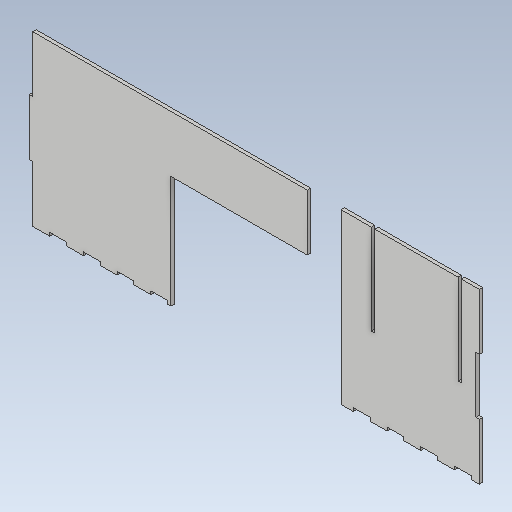
# Autodesk Inventor part: ParedFrontal
Saved by Autodesk Inventor 2020 (Build 240168000, 168)
## iProperties
Created: 2020-03-08
Part Number: ParedFrontal
Material: Genérico
Document SubType Name: Modeling
Designer: Diego Guillén
Density: 1 g/cm^3
Appearance: Valor por defecto
Author: Diego Guillén
Autodesk Inventor part; units mm, degrees
ref_plane "YZ Plane" through (0, 0, 0) normal (1, 0, 0) x (0, 1, 0)
ref_plane "XZ Plane" through (0, 0, 0) normal (0, 1, 0) x (-1, 0, 0)
ref_plane "XY Plane" through (0, 0, 0) normal (0, 0, 1) x (1, 0, 0)
sketch "Boceto1" plane through (0, 0, 0) normal (0, 0, 1) x (1, 0, 0)
  line L0 (0, 0) -> (400, 0)
  line L1 (400, 0) -> (400, 150)
  line L2 (400, 150) -> (0, 150)
  line L3 (0, 150) -> (0, 0)
  dimension "d0" = 150
  dimension "d1" = 400
  constraints: 8 end point, 2 parallel, 1 horizontal, 1 perpendicular
  measures "d0" distance of L0.end L1.end
  measures "d1" distance of L1.end L2.end
extrude "Extrusión1" add sketch "Boceto1" along normal blind 3
sketch "Boceto3" plane through (0, 0, 3) normal (0, 0, 1) x (1, 0, 0)
  line L0 (0, 0) -> (400, 0) construction
  line L1 (400, 0) -> (400, 150) construction
  line L2 (400, 150) -> (0, 150) construction
  line L3 (0, 150) -> (0, 0) construction
  line L4 (0, 50) -> (3, 50)
  line L5 (3, 50) -> (3, 0)
  line L6 (3, 0) -> (0, 0)
  line L7 (0, 0) -> (0, 50)
  line L8 (0, 100) -> (0, 150)
  line L9 (0, 150) -> (3, 150)
  line L10 (3, 150) -> (3, 100)
  line L11 (3, 100) -> (0, 100)
  line L12 (397, 100) -> (400, 100)
  line L13 (400, 100) -> (400, 50)
  line L14 (400, 50) -> (397, 50)
  line L15 (397, 50) -> (397, 100)
  line L16 (400, 0) -> (400, 150) construction
  point P0 (400, 75)
  point P1 (400, 75)
  dimension "d15" = 3
  dimension "d16" = 50
  dimension "d19" = 100
  dimension "d24" = 3
  dimension "d25" = 50
  constraints: 24 end point, 4 parallel, 2 coincident, 2 horizontal, 2 midpoint, 2 perpendicular, 1 collinear, 1 vertical, 8 other
  measures "d15" distance of L5.end L6.end
  measures "d16" distance of L4.end L5.end
  measures "d19" distance of L6.end L8.start
  measures "d24" distance of L13.end L14.end
  measures "d25" distance of L14.end L12.start
extrude "Extrusión3" cut sketch "Boceto3" against normal blind 3
sketch "Boceto4" plane through (0, 0, 3) normal (0, 0, 1) x (1, 0, 0)
  line L0 (3, 150) -> (3, 100) construction
  line L1 (3, 100) -> (0, 100) construction
  line L2 (0, 100) -> (0, 50) construction
  line L3 (0, 50) -> (3, 50) construction
  line L4 (3, 50) -> (3, 0) construction
  line L5 (3, 0) -> (400, 0) construction
  line L6 (400, 0) -> (400, 50) construction
  line L7 (400, 50) -> (397, 50) construction
  line L8 (397, 50) -> (397, 100) construction
  line L9 (397, 100) -> (400, 100) construction
  line L10 (400, 100) -> (400, 150) construction
  line L11 (400, 150) -> (3, 150) construction
  line L12 (277.1, 100) -> (125.9, 100)
  line L13 (125.9, 100) -> (125.9, 0)
  line L14 (125.9, 0) -> (277.1, 0)
  line L15 (277.1, 0) -> (277.1, 100)
  line L16 (3, 0) -> (400, 0) construction
  point P0 (0, 0)
  point P1 (201.5, 0)
  point P2 (201.5, 0)
  dimension "d28" = 151.2
  dimension "d29" = 100
  constraints: 8 end point, 2 midpoint, 2 parallel, 1 coincident, 1 collinear, 1 horizontal, 1 perpendicular
  measures "d28" distance of L12.start L12.end
  measures "d29" distance of L14.end L12.start
extrude "Extrusión4" cut sketch "Boceto4" against normal blind 10
sketch "Boceto5" plane through (0, 0, 3) normal (0, 0, 1) x (1, 0, 0)
  line L0 (277.1, 100) -> (277.1, 0) construction
  line L1 (277.1, 0) -> (400, 0) construction
  line L2 (400, 0) -> (400, 50) construction
  line L3 (400, 50) -> (397, 50) construction
  line L4 (397, 50) -> (397, 100) construction
  line L5 (397, 100) -> (400, 100) construction
  line L6 (400, 100) -> (400, 150) construction
  line L7 (400, 150) -> (3, 150) construction
  line L8 (3, 150) -> (3, 100) construction
  line L9 (3, 100) -> (0, 100) construction
  line L10 (0, 100) -> (0, 50) construction
  line L11 (0, 50) -> (3, 50) construction
  line L12 (3, 50) -> (3, 0) construction
  line L13 (3, 0) -> (125.9, 0) construction
  line L14 (125.9, 0) -> (125.9, 100) construction
  line L15 (125.9, 100) -> (277.1, 100) construction
  line L16 (304.1, 150) -> (307.1, 150)
  line L17 (307.1, 150) -> (307.1, 70)
  line L18 (307.1, 70) -> (304.1, 70)
  line L19 (304.1, 70) -> (304.1, 150)
  line L20 (381.1, 150) -> (384.1, 150)
  line L21 (384.1, 150) -> (384.1, 70)
  line L22 (384.1, 70) -> (381.1, 70)
  line L23 (381.1, 70) -> (381.1, 150)
  line L24 (400, 150) -> (3, 150) construction
  point P0 (0, 0)
  dimension "d32" = 3
  dimension "d33" = 3
  dimension "d34" = 74
  dimension "d35" = 27
  dimension "d36" = 80
  dimension "d37" = 80
  constraints: 16 end point, 4 parallel, 2 horizontal, 2 perpendicular, 1 collinear, 1 point on line
  measures "d32" distance of L17.end L18.end
  measures "d33" distance of L21.end L22.end
  measures "d34" distance between parallel lines of L17 L23
  measures "d35" distance between parallel lines of L0 L19
  measures "d36" distance between parallel lines of L7 L18
  measures "d37" distance between parallel lines of L7 L22
extrude "Extrusión5" cut sketch "Boceto5" against normal blind 10
sketch "Boceto6" plane through (0, 0, 3) normal (0, 0, 1) x (1, 0, 0)
  line L0 (307.1, 150) -> (307.1, 70) construction
  line L1 (307.1, 70) -> (304.1, 70) construction
  line L2 (304.1, 70) -> (304.1, 150) construction
  line L3 (304.1, 150) -> (3, 150) construction
  line L4 (3, 150) -> (3, 100) construction
  line L5 (3, 100) -> (0, 100) construction
  line L6 (0, 100) -> (0, 50) construction
  line L7 (0, 50) -> (3, 50) construction
  line L8 (3, 50) -> (3, 0) construction
  line L9 (3, 0) -> (125.9, 0) construction
  line L10 (125.9, 0) -> (125.9, 100) construction
  line L11 (125.9, 100) -> (277.1, 100) construction
  line L12 (277.1, 100) -> (277.1, 0) construction
  line L13 (277.1, 0) -> (400, 0) construction
  line L14 (400, 0) -> (400, 50) construction
  line L15 (400, 50) -> (397, 50) construction
  line L16 (397, 50) -> (397, 100) construction
  line L17 (397, 100) -> (400, 100) construction
  line L18 (400, 100) -> (400, 150) construction
  line L19 (400, 150) -> (384.1, 150) construction
  line L20 (384.1, 150) -> (384.1, 70) construction
  line L21 (384.1, 70) -> (381.1, 70) construction
  line L22 (381.1, 70) -> (381.1, 150) construction
  line L23 (381.1, 150) -> (307.1, 150) construction
  line L24 (277.1, 100) -> (247.1, 100)
  line L25 (247.1, 100) -> (247.1, 150)
  line L26 (247.1, 150) -> (277.1, 150)
  line L27 (277.1, 150) -> (277.1, 100)
  line L28 (125.9, 100) -> (277.1, 100) construction
  line L29 (304.1, 150) -> (3, 150) construction
  line L30 (277.1, 100) -> (277.1, 0) construction
  point P0 (0, 0)
  dimension "d40" = 30
  constraints: 8 end point, 3 collinear, 2 parallel, 1 horizontal, 1 perpendicular
  measures "d40" distance of L24.start L24.end
extrude "Extrusión6" cut sketch "Boceto6" against normal blind 10
sketch "Boceto7" plane through (0, 0, 3) normal (0, 0, 1) x (1, 0, 0)
  line L0 (247.1, 100) -> (247.1, 150) construction
  line L1 (247.1, 150) -> (3, 150) construction
  line L2 (3, 150) -> (3, 100) construction
  line L3 (3, 100) -> (0, 100) construction
  line L4 (0, 100) -> (0, 50) construction
  line L5 (0, 50) -> (3, 50) construction
  line L6 (3, 50) -> (3, 0) construction
  line L7 (3, 0) -> (125.9, 0) construction
  line L8 (125.9, 0) -> (125.9, 100) construction
  line L9 (125.9, 100) -> (247.1, 100) construction
  line L10 (277.1, 150) -> (277.1, 0) construction
  line L11 (277.1, 0) -> (400, 0) construction
  line L12 (400, 0) -> (400, 50) construction
  line L13 (400, 50) -> (397, 50) construction
  line L14 (397, 50) -> (397, 100) construction
  line L15 (397, 100) -> (400, 100) construction
  line L16 (400, 100) -> (400, 150) construction
  line L17 (400, 150) -> (384.1, 150) construction
  line L18 (384.1, 150) -> (384.1, 70) construction
  line L19 (384.1, 70) -> (381.1, 70) construction
  line L20 (381.1, 70) -> (381.1, 150) construction
  line L21 (381.1, 150) -> (307.1, 150) construction
  line L22 (307.1, 150) -> (307.1, 70) construction
  line L23 (307.1, 70) -> (304.1, 70) construction
  line L24 (304.1, 70) -> (304.1, 150) construction
  line L25 (304.1, 150) -> (277.1, 150) construction
  line L26 (18, 3) -> (33, 3)
  line L27 (33, 3) -> (33, 0)
  line L28 (33, 0) -> (18, 0)
  line L29 (18, 0) -> (18, 3)
  line L30 (3, 0) -> (125.9, 0) construction
  line L31 (63, 0) -> (48, 0)
  line L32 (63, 3) -> (63, 0)
  line L33 (48, 3) -> (63, 3)
  line L34 (48, 0) -> (48, 3)
  line L35 (93, 0) -> (78, 0)
  line L36 (93, 3) -> (93, 0)
  line L37 (78, 3) -> (93, 3)
  line L38 (78, 0) -> (78, 3)
  line L39 (123, 0) -> (108, 0)
  line L40 (123, 3) -> (123, 0)
  line L41 (108, 3) -> (123, 3)
  line L42 (108, 0) -> (108, 3)
  line L43 (153, 0) -> (138, 0)
  line L44 (153, 3) -> (153, 0)
  line L45 (138, 3) -> (153, 3)
  line L46 (138, 0) -> (138, 3)
  line L47 (183, 0) -> (168, 0)
  line L48 (183, 3) -> (183, 0)
  line L49 (168, 3) -> (183, 3)
  line L50 (168, 0) -> (168, 3)
  line L51 (213, 0) -> (198, 0)
  line L52 (213, 3) -> (213, 0)
  line L53 (198, 3) -> (213, 3)
  line L54 (198, 0) -> (198, 3)
  line L55 (243, 0) -> (228, 0)
  line L56 (243, 3) -> (243, 0)
  line L57 (228, 3) -> (243, 3)
  line L58 (228, 0) -> (228, 3)
  line L59 (273, 0) -> (258, 0)
  line L60 (273, 3) -> (273, 0)
  line L61 (258, 3) -> (273, 3)
  line L62 (258, 0) -> (258, 3)
  line L63 (303, 0) -> (288, 0)
  line L64 (303, 3) -> (303, 0)
  line L65 (288, 3) -> (303, 3)
  line L66 (288, 0) -> (288, 3)
  line L67 (333, 0) -> (318, 0)
  line L68 (333, 3) -> (333, 0)
  line L69 (318, 3) -> (333, 3)
  line L70 (318, 0) -> (318, 3)
  line L71 (363, 0) -> (348, 0)
  line L72 (363, 3) -> (363, 0)
  line L73 (348, 3) -> (363, 3)
  line L74 (348, 0) -> (348, 3)
  line L75 (393, 0) -> (378, 0)
  line L76 (393, 3) -> (393, 0)
  line L77 (378, 3) -> (393, 3)
  line L78 (378, 0) -> (378, 3)
  point P0 (0, 0)
  dimension "d43" = 15
  dimension "d44" = 3
  dimension "d45" = 15
  dimension "d53" = 30
  constraints: 104 end point, 2 horizontal, 2 parallel, 1 collinear, 1 perpendicular, 96 other
  measures "d43" distance of L26.start L26.end
  measures "d44" distance of L26.end L27.end
  measures "d45" distance between parallel lines of L6 L29
  measures "d53" distance of L27.end L31.start
extrude "Extrusión7" cut sketch "Boceto7" against normal blind 10
